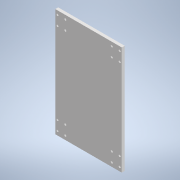
# Autodesk Inventor part: base
Saved by Autodesk Inventor 2022 (Build 260153000, 153)
## iProperties
Created: 2023-05-18
Part Number: base
Material: Типовые
Document SubType Name: Modeling
Designer: Robo0
Density: 1 g/cm^3
Appearance: По умолчанию
Author: Robo0
Autodesk Inventor part; units mm, degrees
ref_plane "YZ Plane" through (0, 0, 0) normal (1, 0, 0) x (0, 1, 0)
ref_plane "XZ Plane" through (0, 0, 0) normal (0, 1, 0) x (-1, 0, 0)
ref_plane "XY Plane" through (0, 0, 0) normal (0, 0, 1) x (1, 0, 0)
sketch "Эскиз1" plane through (0, 0, 0) normal (0, 0, 1) x (1, 0, 0)
  circle A0 centre (-29.5, 10.2953) radius 2 projected
  circle A1 centre (-45.5, 10.2953) radius 2 projected
  circle A2 centre (-45.5, 29.7047) radius 2 projected
  circle A3 centre (-29.5, 29.7047) radius 2 projected
  circle A4 centre (-156.1512, 10.3104) radius 2 projected
  circle A5 centre (-140.1512, 10.3104) radius 2 projected
  circle A6 centre (-140.1512, 29.7197) radius 2 projected
  circle A7 centre (-156.1512, 29.7197) radius 2 projected
  circle A8 centre (-140.1512, 195.7348) radius 2 projected
  circle A9 centre (-156.1512, 195.7348) radius 2 projected
  circle A10 centre (-140.1512, 215.1441) radius 2 projected
  circle A11 centre (-156.1512, 215.1441) radius 2 projected
  circle A12 centre (-29.5, 215.129) radius 2 projected
  circle A13 centre (-29.5, 195.7197) radius 2 projected
  circle A14 centre (-45.5, 195.7197) radius 2 projected
  circle A15 centre (-45.5, 215.129) radius 2 projected
  line L0 (-25, -1.891) -> (-25, 41.891) projected
  line L1 (-11.2, 1) -> (-52.2, 1)
  line L2 (-160.6512, 227.3305) -> (-160.6512, 183.5485) projected
  line L3 (-132.8256, 223.1441) -> (-185.6512, 223.1441) projected
  line L4 (-52.8256, 2.2953) -> (0, 2.2953) projected
  line L5 (-25, 2.2953) -> (-160.6512, 2.2953)
  line L6 (-160.6512, 2.2953) -> (-160.6512, 223.1441)
  line L7 (-160.6512, 223.1441) -> (-25, 223.1441)
  line L8 (-25, 223.1441) -> (-25, 2.2953)
  point P0 (0, 0)
  constraints: 10 end point, 4 point on line, 2 horizontal, 2 parallel, 1 perpendicular, 2 other
extrude "Выдавливание1" add sketch "Эскиз1" along normal blind 6
